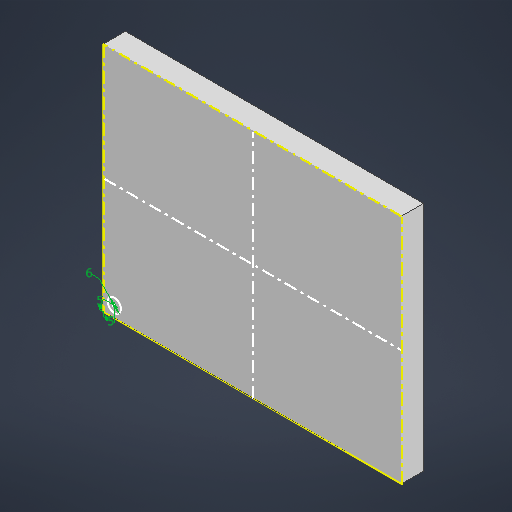
# Autodesk Inventor part: boden
Saved by Autodesk Inventor 2027 (Build 310192060, 192F)
## iProperties
Created: 2026-06-16
Part Number: boden
Material: Generic
Document SubType Name: Modeling
Designer: Felix
Density: 1 g/cm^3
Appearance: Default
Author: Felix
Autodesk Inventor part; units mm, degrees
ref_plane "YZ Plane" through (0, 0, 0) normal (1, 0, 0) x (0, 1, 0)
ref_plane "XZ Plane" through (0, 0, 0) normal (0, 1, 0) x (-1, 0, 0)
ref_plane "XY Plane" through (0, 0, 0) normal (0, 0, 1) x (1, 0, 0)
sketch "Sketch3" plane through (0, 0, 0) normal (0, 0, 1) x (1, 0, 0)
  line L0 (0, 0) -> (135, 0)
  line L1 (135, 0) -> (135, 105)
  line L2 (135, 105) -> (0, 105)
  line L3 (0, 105) -> (0, 0)
  dimension "d24" = 135
  dimension "d25" = 105
  constraints: 8 end point, 2 parallel, 1 horizontal, 1 perpendicular
  measures "d24" distance of L2.end L1.end
  measures "d25" distance of L1.end L0.end
extrude "Extrusion1" add sketch "Sketch3" along normal blind 10
sketch "Sketch1" plane through (0, 0, 0) normal (0, 0, 1) x (1, 0, 0)
  circle A0 centre (5, 33) radius 2
  circle A1 centre (52, 33) radius 2
  circle A2 centre (5, 10) radius 2
  circle A3 centre (10, 85) radius 2
  circle A4 centre (68, 85) radius 2
  circle A5 centre (10, 53) radius 2
  circle A6 centre (87, 46.9) radius 2
  circle A7 centre (123.9, 46.9) radius 2
  circle A8 centre (87, 10) radius 2
  point P0 (0, 0)
  point P1 (3.899, 77.9301)
  dimension "d0" = 4
  dimension "d1" = 4
  dimension "d2" = 4
  dimension "d3" = 23
  dimension "d4" = 47
  dimension "d6" = 4
  dimension "d7" = 4
  dimension "d8" = 4
  dimension "d9" = 32
  dimension "d10" = 58
  dimension "d11" = 5
  dimension "d12" = 20
  dimension "d13" = 4
  dimension "d14" = 4
  dimension "d15" = 4
  dimension "d16" = 36.9
  dimension "d17" = 36.9
  dimension "d18" = 35
  dimension "d28" = 10
  dimension "d29" = 5
  constraints: 9 centre point, 4 horizontal alignment, 3 vertical alignment
  measures "d0" diameter of A0
  measures "d1" diameter of A1
  measures "d2" diameter of A2
  measures "d3" distance of A2.centre A0.centre
  measures "d4" distance of A1.centre A0.centre
  measures "d6" diameter of A3
  measures "d7" diameter of A4
  measures "d8" diameter of A5
  measures "d9" distance of A5.centre A3.centre
  measures "d10" distance of A4.centre A3.centre
  measures "d11" horizontal distance of A0.centre A5.centre
  measures "d12" vertical distance of A0.centre A5.centre
  measures "d13" diameter of A6
  measures "d14" diameter of A7
  measures "d15" diameter of A8
  measures "d16" distance of A8.centre A6.centre
  measures "d17" distance of A7.centre A6.centre
  measures "d18" horizontal distance of A8.centre A1.centre
  measures "d28" vertical distance of point (0, 0) A2.centre
  measures "d29" horizontal distance of point (0, 0) A2.centre
extrude "Extrusion2" cut sketch "Sketch1" along normal blind 5.7
sketch "Sketch4" plane through (0, 0, 10) normal (0, 0, 1) x (1, 0, 0)
  circle A0 centre (5, 5) radius 3
  line L0 (0, 105) -> (0, 0) projected
  line L1 (0, 0) -> (135, 0) projected
  line L2 (0, 105) -> (0, 0) projected
  line L3 (0, 52.5) -> (135, 52.5)
  line L4 (135, 0) -> (135, 105) projected
  line L5 (67.5, 0) -> (67.5, 105)
  line L6 (135, 105) -> (0, 105) projected
  dimension "d32" = 6
  dimension "d33" = 5
  dimension "d34" = 5
  constraints: 4 end point, 4 midpoint, 1 centre point
  measures "d32" diameter of A0
  measures "d33" distance from line of L0 A0.centre
  measures "d34" distance from line of L1 A0.centre
body "Solid1"
